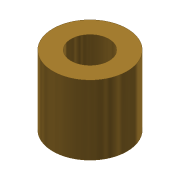
# Autodesk Inventor part: shaft plane bushes
Saved by Autodesk Inventor 2015 (Build 190159000, 159)
## iProperties
Created: 2020-03-27
Part Number: shaft plane bushes
Material: Brass, Soft Yellow
Document SubType Name: Modeling
Designer: Ghassan Yusuf
Density: 8.47 g/cm^3
Appearance: Brass - Satin
Author: Ghassan Yusuf
Autodesk Inventor part; units mm, degrees
ref_plane "YZ Plane" through (0, 0, 0) normal (1, 0, 0) x (0, 1, 0)
ref_plane "XZ Plane" through (0, 0, 0) normal (0, 1, 0) x (-1, 0, 0)
ref_plane "XY Plane" through (0, 0, 0) normal (0, 0, 1) x (1, 0, 0)
sketch "Sketch1" plane through (0, 0, 0) normal (0, 0, 1) x (1, 0, 0)
  circle A0 centre (0, 0) radius 8
  circle A1 centre (0, 0) radius 4.1
  dimension "d0" = 16
  dimension "d1" = 8.2
  constraints: 2 centre point, 2 coincident
  measures "d0" diameter of A0
  measures "d1" diameter of A1
extrude "Extrusion1" add sketch "Sketch1" along normal mid plane 15
body "Solid1"
